Autodesk Fusion 360 part; units mm, degrees
(part 5 of 6)
  arc A937 (93.55, -32.3196) -> (93.5061, -32.1633) centre (93.25, -32.3196) ccw
  arc A938 (94.1933, -31.4761) -> (93.5061, -32.1633) centre (93.9328, -31.9028) ccw
  arc A939 (94.1933, -31.4761) -> (94.3496, -31.52) centre (94.3496, -31.22) ccw
  line L528 (94.3496, -31.52) -> (95.25, -31.52)
  line L529 (95.25, -31.52) -> (96.1504, -31.52)
  arc A940 (96.1504, -31.52) -> (96.3067, -31.4761) centre (96.1503, -31.22) ccw
  arc A941 (96.9939, -32.1633) -> (96.3067, -31.4761) centre (96.5672, -31.9028) ccw
  arc A942 (96.9939, -32.1633) -> (96.95, -32.3196) centre (97.2501, -32.3197) ccw
  line L530 (96.95, -32.3196) -> (96.95, -33.02)
  line L531 (96.95, -33.02) -> (96.95, -33.7204)
  arc A943 (96.95, -33.7204) -> (96.9939, -33.8767) centre (97.25, -33.7203) ccw
  circle A944 centre (78.4225, -19.3675) radius 1.5
  circle A945 centre (59.3725, -19.3675) radius 1.5
  arc A946 (77.2567, -34.5639) -> (77.9439, -33.8767) centre (77.5172, -34.1372) ccw
  arc A947 (77.2567, -34.5639) -> (77.1004, -34.52) centre (77.1004, -34.8197) ccw
  line L532 (77.1004, -34.52) -> (76.2, -34.52)
  line L533 (76.2, -34.52) -> (75.2996, -34.52)
  arc A948 (75.2996, -34.52) -> (75.1433, -34.5639) centre (75.2996, -34.82) ccw
  arc A949 (74.4561, -33.8767) -> (75.1433, -34.5639) centre (74.8828, -34.1372) ccw
  arc A950 (74.4561, -33.8767) -> (74.5, -33.7204) centre (74.2, -33.7204) ccw
  line L534 (74.5, -33.7204) -> (74.5, -33.02)
  line L535 (74.5, -33.02) -> (74.5, -32.3196)
  arc A951 (74.5, -32.3196) -> (74.4561, -32.1633) centre (74.2, -32.3196) ccw
  arc A952 (75.1433, -31.4761) -> (74.4561, -32.1633) centre (74.8828, -31.9028) ccw
  arc A953 (75.1433, -31.4761) -> (75.2996, -31.52) centre (75.2996, -31.22) ccw
  line L536 (75.2996, -31.52) -> (76.2, -31.52)
  line L537 (76.2, -31.52) -> (77.1004, -31.52)
  arc A954 (77.1004, -31.52) -> (77.2567, -31.4761) centre (77.1003, -31.22) ccw
  arc A955 (77.9439, -32.1633) -> (77.2567, -31.4761) centre (77.5172, -31.9028) ccw
  arc A956 (77.9439, -32.1633) -> (77.9, -32.3196) centre (78.2001, -32.3197) ccw
  line L538 (77.9, -32.3196) -> (77.9, -33.02)
  line L539 (77.9, -33.02) -> (77.9, -33.7204)
  arc A957 (77.9, -33.7204) -> (77.9439, -33.8767) centre (78.2, -33.7203) ccw
  arc A958 (58.2067, -34.5639) -> (58.8939, -33.8767) centre (58.4672, -34.1372) ccw
  arc A959 (58.2067, -34.5639) -> (58.0504, -34.52) centre (58.0504, -34.8197) ccw
  line L540 (58.0504, -34.52) -> (57.15, -34.52)
  line L541 (57.15, -34.52) -> (56.2496, -34.52)
  arc A960 (56.2496, -34.52) -> (56.0933, -34.5639) centre (56.2496, -34.82) ccw
  arc A961 (55.4061, -33.8767) -> (56.0933, -34.5639) centre (55.8328, -34.1372) ccw
  arc A962 (55.4061, -33.8767) -> (55.45, -33.7204) centre (55.15, -33.7204) ccw
  line L542 (55.45, -33.7204) -> (55.45, -33.02)
  line L543 (55.45, -33.02) -> (55.45, -32.3196)
  arc A963 (55.45, -32.3196) -> (55.4061, -32.1633) centre (55.15, -32.3196) ccw
  arc A964 (56.0933, -31.4761) -> (55.4061, -32.1633) centre (55.8328, -31.9028) ccw
  arc A965 (56.0933, -31.4761) -> (56.2496, -31.52) centre (56.2496, -31.22) ccw
  line L544 (56.2496, -31.52) -> (57.15, -31.52)
  line L545 (57.15, -31.52) -> (58.0504, -31.52)
  arc A966 (58.0504, -31.52) -> (58.2067, -31.4761) centre (58.0503, -31.22) ccw
  arc A967 (58.8939, -32.1633) -> (58.2067, -31.4761) centre (58.4672, -31.9028) ccw
  arc A968 (58.8939, -32.1633) -> (58.85, -32.3196) centre (59.1501, -32.3197) ccw
  line L546 (58.85, -32.3196) -> (58.85, -33.02)
  line L547 (58.85, -33.02) -> (58.85, -33.7204)
  arc A969 (58.85, -33.7204) -> (58.8939, -33.8767) centre (59.15, -33.7203) ccw
  circle A970 centre (124.1425, -38.1) radius 0.875
  circle A971 centre (122.8725, -40.64) radius 1.5
  circle A972 centre (119.0625, -38.1) radius 1.9939
  circle A973 centre (113.9825, -38.1) radius 0.875
  circle A974 centre (100.33, -38.1) radius 0.875
  circle A975 centre (95.25, -38.1) radius 1.9939
  circle A976 centre (90.17, -38.1) radius 0.875
  circle A977 centre (99.06, -40.64) radius 1.5
  circle A978 centre (116.5225, -43.18) radius 1.5
  circle A979 centre (128.5875, -47.625) radius 1.1
  circle A980 centre (92.71, -43.18) radius 1.5
  circle A981 centre (107.1563, -47.625) radius 1.1
  circle A982 centre (81.28, -38.1) radius 0.875
  circle A983 centre (76.2, -38.1) radius 1.9939
  circle A984 centre (71.12, -38.1) radius 0.875
  circle A985 centre (80.01, -40.64) radius 1.5
  circle A986 centre (62.23, -38.1) radius 0.875
  circle A987 centre (60.96, -40.64) radius 1.5
  circle A988 centre (57.15, -38.1) radius 1.9939
  circle A989 centre (52.07, -38.1) radius 0.875
  circle A990 centre (73.66, -43.18) radius 1.5
  circle A991 centre (54.61, -43.18) radius 1.5
  circle A992 centre (40.3225, -19.3675) radius 1.5
  circle A993 centre (21.2725, -19.3675) radius 1.5
  arc A994 (39.1567, -34.5639) -> (39.8439, -33.8767) centre (39.4172, -34.1372) ccw
  arc A995 (39.1567, -34.5639) -> (39.0004, -34.52) centre (39.0004, -34.8197) ccw
  line L548 (39.0004, -34.52) -> (38.1, -34.52)
  line L549 (38.1, -34.52) -> (37.1996, -34.52)
  arc A996 (37.1996, -34.52) -> (37.0433, -34.5639) centre (37.1996, -34.82) ccw
  arc A997 (36.3561, -33.8767) -> (37.0433, -34.5639) centre (36.7828, -34.1372) ccw
  arc A998 (36.3561, -33.8767) -> (36.4, -33.7204) centre (36.1, -33.7204) ccw
  line L550 (36.4, -33.7204) -> (36.4, -33.02)
  line L551 (36.4, -33.02) -> (36.4, -32.3196)
  arc A999 (36.4, -32.3196) -> (36.3561, -32.1633) centre (36.1, -32.3196) ccw
  arc A1000 (37.0433, -31.4761) -> (36.3561, -32.1633) centre (36.7828, -31.9028) ccw
  arc A1001 (37.0433, -31.4761) -> (37.1996, -31.52) centre (37.1996, -31.22) ccw
  line L552 (37.1996, -31.52) -> (38.1, -31.52)
  line L553 (38.1, -31.52) -> (39.0004, -31.52)
  arc A1002 (39.0004, -31.52) -> (39.1567, -31.4761) centre (39.0003, -31.22) ccw
  arc A1003 (39.8439, -32.1633) -> (39.1567, -31.4761) centre (39.4172, -31.9028) ccw
  arc A1004 (39.8439, -32.1633) -> (39.8, -32.3196) centre (40.1001, -32.3197) ccw
  line L554 (39.8, -32.3196) -> (39.8, -33.02)
  line L555 (39.8, -33.02) -> (39.8, -33.7204)
  arc A1005 (39.8, -33.7204) -> (39.8439, -33.8767) centre (40.1, -33.7203) ccw
  circle A1006 centre (26.1938, -26.1938) radius 1.1
  arc A1007 (15.3442, -34.5639) -> (16.0314, -33.8767) centre (15.6047, -34.1372) ccw
  arc A1008 (15.3442, -34.5639) -> (15.1879, -34.52) centre (15.1879, -34.8197) ccw
  line L556 (15.1879, -34.52) -> (14.2875, -34.52)
  line L557 (14.2875, -34.52) -> (13.3871, -34.52)
  arc A1009 (13.3871, -34.52) -> (13.2308, -34.5639) centre (13.3871, -34.82) ccw
  arc A1010 (12.5436, -33.8767) -> (13.2308, -34.5639) centre (12.9703, -34.1372) ccw
  arc A1011 (12.5436, -33.8767) -> (12.5875, -33.7204) centre (12.2875, -33.7204) ccw
  line L558 (12.5875, -33.7204) -> (12.5875, -33.02)
  line L559 (12.5875, -33.02) -> (12.5875, -32.3196)
  arc A1012 (12.5875, -32.3196) -> (12.5436, -32.1633) centre (12.2875, -32.3196) ccw
  arc A1013 (13.2308, -31.4761) -> (12.5436, -32.1633) centre (12.9703, -31.9028) ccw
  arc A1014 (13.2308, -31.4761) -> (13.3871, -31.52) centre (13.3871, -31.22) ccw
  line L560 (13.3871, -31.52) -> (14.2875, -31.52)
  line L561 (14.2875, -31.52) -> (15.1879, -31.52)
  arc A1015 (15.1879, -31.52) -> (15.3442, -31.4761) centre (15.1878, -31.22) ccw
  arc A1016 (16.0314, -32.1633) -> (15.3442, -31.4761) centre (15.6047, -31.9028) ccw
  arc A1017 (16.0314, -32.1633) -> (15.9875, -32.3196) centre (16.2876, -32.3197) ccw
  line L562 (15.9875, -32.3196) -> (15.9875, -33.02)
  line L563 (15.9875, -33.02) -> (15.9875, -33.7204)
  arc A1018 (15.9875, -33.7204) -> (16.0314, -33.8767) centre (16.2875, -33.7203) ccw
  circle A1019 centre (2.2225, -19.3675) radius 1.5
  circle A1020 centre (-16.8275, -19.3675) radius 1.5
  arc A1021 (-6.5064, -33.8767) -> (-5.8192, -34.5639) centre (-6.0797, -34.1372) ccw
  arc A1022 (-6.5064, -33.8767) -> (-6.4625, -33.7204) centre (-6.7625, -33.7204) ccw
  line L564 (-6.4625, -33.7204) -> (-6.4625, -33.02)
  line L565 (-6.4625, -33.02) -> (-6.4625, -32.3196)
  arc A1023 (-6.4625, -32.3196) -> (-6.5064, -32.1633) centre (-6.7625, -32.3196) ccw
  arc A1024 (-5.8192, -31.4761) -> (-6.5064, -32.1633) centre (-6.0797, -31.9028) ccw
  arc A1025 (-5.8192, -31.4761) -> (-5.6629, -31.52) centre (-5.6629, -31.22) ccw
  line L566 (-5.6629, -31.52) -> (-4.7625, -31.52)
  line L567 (-4.7625, -31.52) -> (-3.8621, -31.52)
  arc A1026 (-3.8621, -31.52) -> (-3.7058, -31.4761) centre (-3.8622, -31.22) ccw
  arc A1027 (-3.0186, -32.1633) -> (-3.7058, -31.4761) centre (-3.4453, -31.9028) ccw
  arc A1028 (-3.0186, -32.1633) -> (-3.0625, -32.3196) centre (-2.7624, -32.3197) ccw
  line L568 (-3.0625, -32.3196) -> (-3.0625, -33.02)
  line L569 (-3.0625, -33.02) -> (-3.0625, -33.7204)
  arc A1029 (-3.0625, -33.7204) -> (-3.0186, -33.8767) centre (-2.7625, -33.7203) ccw
  arc A1030 (-3.7058, -34.5639) -> (-3.0186, -33.8767) centre (-3.4453, -34.1372) ccw
  arc A1031 (-3.7058, -34.5639) -> (-3.8621, -34.52) centre (-3.8621, -34.8197) ccw
  line L570 (-3.8621, -34.52) -> (-4.7625, -34.52)
  line L571 (-4.7625, -34.52) -> (-5.6629, -34.52)
  arc A1032 (-5.6629, -34.52) -> (-5.8192, -34.5639) centre (-5.6629, -34.82) ccw
  arc A1033 (-25.5564, -33.8767) -> (-24.8692, -34.5639) centre (-25.1297, -34.1372) ccw
  arc A1034 (-25.5564, -33.8767) -> (-25.5125, -33.7204) centre (-25.8125, -33.7204) ccw
  line L572 (-25.5125, -33.7204) -> (-25.5125, -33.02)
  line L573 (-25.5125, -33.02) -> (-25.5125, -32.3196)
  arc A1035 (-25.5125, -32.3196) -> (-25.5564, -32.1633) centre (-25.8125, -32.3196) ccw
  arc A1036 (-24.8692, -31.4761) -> (-25.5564, -32.1633) centre (-25.1297, -31.9028) ccw
  arc A1037 (-24.8692, -31.4761) -> (-24.7129, -31.52) centre (-24.7129, -31.22) ccw
  line L574 (-24.7129, -31.52) -> (-23.8125, -31.52)
  line L575 (-23.8125, -31.52) -> (-22.9121, -31.52)
  arc A1038 (-22.9121, -31.52) -> (-22.7558, -31.4761) centre (-22.9122, -31.22) ccw
  arc A1039 (-22.0686, -32.1633) -> (-22.7558, -31.4761) centre (-22.4953, -31.9028) ccw
  arc A1040 (-22.0686, -32.1633) -> (-22.1125, -32.3196) centre (-21.8124, -32.3197) ccw
  line L576 (-22.1125, -32.3196) -> (-22.1125, -33.02)
  line L577 (-22.1125, -33.02) -> (-22.1125, -33.7204)
  arc A1041 (-22.1125, -33.7204) -> (-22.0686, -33.8767) centre (-21.8125, -33.7203) ccw
  arc A1042 (-22.7558, -34.5639) -> (-22.0686, -33.8767) centre (-22.4953, -34.1372) ccw
  arc A1043 (-22.7558, -34.5639) -> (-22.9121, -34.52) centre (-22.9121, -34.8197) ccw
  line L578 (-22.9121, -34.52) -> (-23.8125, -34.52)
  line L579 (-23.8125, -34.52) -> (-24.7129, -34.52)
  arc A1044 (-24.7129, -34.52) -> (-24.8692, -34.5639) centre (-24.7129, -34.82) ccw
  circle A1045 centre (43.18, -38.1) radius 0.875
  circle A1046 centre (41.91, -40.64) radius 1.5
  circle A1047 centre (38.1, -38.1) radius 1.9939
  circle A1048 centre (33.02, -38.1) radius 0.875
  circle A1049 centre (19.3675, -38.1) radius 0.875
  circle A1050 centre (14.2875, -38.1) radius 1.9939
  circle A1051 centre (18.0975, -40.64) radius 1.5
  circle A1052 centre (35.56, -43.18) radius 1.5
  circle A1053 centre (11.7475, -43.18) radius 1.5
  circle A1054 centre (26.1938, -47.625) radius 1.1
  circle A1055 centre (9.2075, -38.1) radius 0.875
  circle A1056 centre (0.3175, -38.1) radius 0.875
  circle A1057 centre (-4.7625, -38.1) radius 1.9939
  circle A1058 centre (-0.9525, -40.64) radius 1.5
  circle A1059 centre (-9.8425, -38.1) radius 0.875
  circle A1060 centre (-18.7325, -38.1) radius 0.875
  circle A1061 centre (-23.8125, -38.1) radius 1.9939
  circle A1062 centre (-20.0025, -40.64) radius 1.5
  circle A1063 centre (-7.3025, -43.18) radius 1.5
  circle A1064 centre (-26.3525, -43.18) radius 1.5
  arc A1065 (-44.6064, 8.9858) -> (-43.9192, 8.2986) centre (-44.1797, 8.7253) ccw
  arc A1066 (-44.6064, 8.9858) -> (-44.5625, 9.1421) centre (-44.8625, 9.1421) ccw
  line L580 (-44.5625, 9.1421) -> (-44.5625, 9.8425)
  line L581 (-44.5625, 9.8425) -> (-44.5625, 10.5429)
  arc A1067 (-44.5625, 10.5429) -> (-44.6064, 10.6992) centre (-44.8625, 10.5429) ccw
  arc A1068 (-43.9192, 11.3864) -> (-44.6064, 10.6992) centre (-44.1797, 10.9597) ccw
  arc A1069 (-43.9192, 11.3864) -> (-43.7629, 11.3425) centre (-43.7629, 11.6425) ccw
  line L582 (-43.7629, 11.3425) -> (-42.8625, 11.3425)
  line L583 (-42.8625, 11.3425) -> (-41.9621, 11.3425)
  arc A1070 (-41.9621, 11.3425) -> (-41.8058, 11.3864) centre (-41.9622, 11.6425) ccw
  arc A1071 (-41.1186, 10.6992) -> (-41.8058, 11.3864) centre (-41.5453, 10.9597) ccw
  arc A1072 (-41.1186, 10.6992) -> (-41.1625, 10.5429) centre (-40.8624, 10.5428) ccw
  line L584 (-41.1625, 10.5429) -> (-41.1625, 9.8425)
  line L585 (-41.1625, 9.8425) -> (-41.1625, 9.1421)
  arc A1073 (-41.1625, 9.1421) -> (-41.1186, 8.9858) centre (-40.8625, 9.1422) ccw
  arc A1074 (-41.8058, 8.2986) -> (-41.1186, 8.9858) centre (-41.5453, 8.7253) ccw
  arc A1075 (-41.8058, 8.2986) -> (-41.9621, 8.3425) centre (-41.9621, 8.0428) ccw
  line L586 (-41.9621, 8.3425) -> (-42.8625, 8.3425)
  line L587 (-42.8625, 8.3425) -> (-43.7629, 8.3425)
  arc A1076 (-43.7629, 8.3425) -> (-43.9192, 8.2986) centre (-43.7629, 8.0425) ccw
  arc A1077 (-63.6564, 8.9858) -> (-62.9692, 8.2986) centre (-63.2297, 8.7253) ccw
  arc A1078 (-63.6564, 8.9858) -> (-63.6125, 9.1421) centre (-63.9125, 9.1421) ccw
  line L588 (-63.6125, 9.1421) -> (-63.6125, 9.8425)
  line L589 (-63.6125, 9.8425) -> (-63.6125, 10.5429)
  arc A1079 (-63.6125, 10.5429) -> (-63.6564, 10.6992) centre (-63.9125, 10.5429) ccw
  arc A1080 (-62.9692, 11.3864) -> (-63.6564, 10.6992) centre (-63.2297, 10.9597) ccw
  arc A1081 (-62.9692, 11.3864) -> (-62.8129, 11.3425) centre (-62.8129, 11.6425) ccw
  line L590 (-62.8129, 11.3425) -> (-61.9125, 11.3425)
  line L591 (-61.9125, 11.3425) -> (-61.0121, 11.3425)
  arc A1082 (-61.0121, 11.3425) -> (-60.8558, 11.3864) centre (-61.0122, 11.6425) ccw
  arc A1083 (-60.1686, 10.6992) -> (-60.8558, 11.3864) centre (-60.5953, 10.9597) ccw
  arc A1084 (-60.1686, 10.6992) -> (-60.2125, 10.5429) centre (-59.9124, 10.5428) ccw
  line L592 (-60.2125, 10.5429) -> (-60.2125, 9.8425)
  line L593 (-60.2125, 9.8425) -> (-60.2125, 9.1421)
  arc A1085 (-60.2125, 9.1421) -> (-60.1686, 8.9858) centre (-59.9125, 9.1422) ccw
  arc A1086 (-60.8558, 8.2986) -> (-60.1686, 8.9858) centre (-60.5953, 8.7253) ccw
  arc A1087 (-60.8558, 8.2986) -> (-61.0121, 8.3425) centre (-61.0121, 8.0428) ccw
  line L594 (-61.0121, 8.3425) -> (-61.9125, 8.3425)
  line L595 (-61.9125, 8.3425) -> (-62.8129, 8.3425)
  arc A1088 (-62.8129, 8.3425) -> (-62.9692, 8.2986) centre (-62.8129, 8.0425) ccw
  circle A1089 centre (-28.8925, 4.7625) radius 0.875
  circle A1090 centre (-37.7825, 4.7625) radius 0.875
  circle A1091 centre (-42.8625, 4.7625) radius 1.9939
  circle A1092 centre (-47.9425, 4.7625) radius 0.875
  circle A1093 centre (-39.0525, 2.2225) radius 1.5
  circle A1094 centre (-45.4025, -0.3175) radius 1.5
  circle A1095 centre (-56.8325, 4.7625) radius 0.875
  circle A1096 centre (-58.1025, 2.2225) radius 1.5
  circle A1097 centre (-61.9125, 4.7625) radius 1.9939
  circle A1098 centre (-66.9925, 4.7625) radius 0.875
  circle A1099 centre (-64.4525, -0.3175) radius 1.5
  arc A1100 (-82.7064, 8.9858) -> (-82.0192, 8.2986) centre (-82.2797, 8.7253) ccw
  arc A1101 (-82.7064, 8.9858) -> (-82.6625, 9.1421) centre (-82.9625, 9.1421) ccw
  line L596 (-82.6625, 9.1421) -> (-82.6625, 9.8425)
  line L597 (-82.6625, 9.8425) -> (-82.6625, 10.5429)
  arc A1102 (-82.6625, 10.5429) -> (-82.7064, 10.6992) centre (-82.9625, 10.5429) ccw
  arc A1103 (-82.0192, 11.3864) -> (-82.7064, 10.6992) centre (-82.2797, 10.9597) ccw
  arc A1104 (-82.0192, 11.3864) -> (-81.8629, 11.3425) centre (-81.8629, 11.6425) ccw
  line L598 (-81.8629, 11.3425) -> (-80.9625, 11.3425)
  line L599 (-80.9625, 11.3425) -> (-80.0621, 11.3425)
  arc A1105 (-80.0621, 11.3425) -> (-79.9058, 11.3864) centre (-80.0622, 11.6425) ccw
  arc A1106 (-79.2186, 10.6992) -> (-79.9058, 11.3864) centre (-79.6453, 10.9597) ccw
  arc A1107 (-79.2186, 10.6992) -> (-79.2625, 10.5429) centre (-78.9624, 10.5428) ccw
  line L600 (-79.2625, 10.5429) -> (-79.2625, 9.8425)
  line L601 (-79.2625, 9.8425) -> (-79.2625, 9.1421)
  arc A1108 (-79.2625, 9.1421) -> (-79.2186, 8.9858) centre (-78.9625, 9.1422) ccw
  arc A1109 (-79.9058, 8.2986) -> (-79.2186, 8.9858) centre (-79.6453, 8.7253) ccw
  arc A1110 (-79.9058, 8.2986) -> (-80.0621, 8.3425) centre (-80.0621, 8.0428) ccw
  line L602 (-80.0621, 8.3425) -> (-80.9625, 8.3425)
  line L603 (-80.9625, 8.3425) -> (-81.8629, 8.3425)
  arc A1111 (-81.8629, 8.3425) -> (-82.0192, 8.2986) centre (-81.8629, 8.0425) ccw
  arc A1112 (-101.7564, 8.9858) -> (-101.0692, 8.2986) centre (-101.3297, 8.7253) ccw
  arc A1113 (-101.7564, 8.9858) -> (-101.7125, 9.1421) centre (-102.0125, 9.1421) ccw
  line L604 (-101.7125, 9.1421) -> (-101.7125, 9.8425)
  line L605 (-101.7125, 9.8425) -> (-101.7125, 10.5429)
  arc A1114 (-101.7125, 10.5429) -> (-101.7564, 10.6992) centre (-102.0125, 10.5429) ccw
  arc A1115 (-101.0692, 11.3864) -> (-101.7564, 10.6992) centre (-101.3297, 10.9597) ccw
  arc A1116 (-101.0692, 11.3864) -> (-100.9129, 11.3425) centre (-100.9129, 11.6425) ccw
  line L606 (-100.9129, 11.3425) -> (-100.0125, 11.3425)
  line L607 (-100.0125, 11.3425) -> (-99.1121, 11.3425)
  arc A1117 (-99.1121, 11.3425) -> (-98.9558, 11.3864) centre (-99.1122, 11.6425) ccw
  arc A1118 (-98.2686, 10.6992) -> (-98.9558, 11.3864) centre (-98.6953, 10.9597) ccw
  arc A1119 (-98.2686, 10.6992) -> (-98.3125, 10.5429) centre (-98.0124, 10.5428) ccw
  line L608 (-98.3125, 10.5429) -> (-98.3125, 9.8425)
  line L609 (-98.3125, 9.8425) -> (-98.3125, 9.1421)
  arc A1120 (-98.3125, 9.1421) -> (-98.2686, 8.9858) centre (-98.0125, 9.1422) ccw
  arc A1121 (-98.9558, 8.2986) -> (-98.2686, 8.9858) centre (-98.6953, 8.7253) ccw
  arc A1122 (-98.9558, 8.2986) -> (-99.1121, 8.3425) centre (-99.1121, 8.0428) ccw
  line L610 (-99.1121, 8.3425) -> (-100.0125, 8.3425)
  line L611 (-100.0125, 8.3425) -> (-100.9129, 8.3425)
  arc A1123 (-100.9129, 8.3425) -> (-101.0692, 8.2986) centre (-100.9129, 8.0425) ccw
  circle A1124 centre (-75.8825, 4.7625) radius 0.875
  circle A1125 centre (-77.1525, 2.2225) radius 1.5
  circle A1126 centre (-80.9625, 4.7625) radius 1.9939
  circle A1127 centre (-86.0425, 4.7625) radius 0.875
  circle A1128 centre (-83.5025, -0.3175) radius 1.5
  circle A1129 centre (-94.9325, 4.7625) radius 0.875
  circle A1130 centre (-96.2025, 2.2225) radius 1.5
  circle A1131 centre (-100.0125, 4.7625) radius 1.9939
  circle A1132 centre (-105.0925, 4.7625) radius 0.875
  circle A1133 centre (-102.5525, -0.3175) radius 1.5
  arc A1134 (-35.0814, -10.0642) -> (-34.3942, -10.7514) centre (-34.6547, -10.3247) ccw
  arc A1135 (-35.0814, -10.0642) -> (-35.0375, -9.9079) centre (-35.3375, -9.9079) ccw
  line L612 (-35.0375, -9.9079) -> (-35.0375, -9.2075)
  line L613 (-35.0375, -9.2075) -> (-35.0375, -8.5071)
  arc A1136 (-35.0375, -8.5071) -> (-35.0814, -8.3508) centre (-35.3375, -8.5071) ccw
  arc A1137 (-34.3942, -7.6636) -> (-35.0814, -8.3508) centre (-34.6547, -8.0903) ccw
  arc A1138 (-34.3942, -7.6636) -> (-34.2379, -7.7075) centre (-34.2379, -7.4075) ccw
  line L614 (-34.2379, -7.7075) -> (-33.3375, -7.7075)
  line L615 (-33.3375, -7.7075) -> (-32.4371, -7.7075)
  arc A1139 (-32.4371, -7.7075) -> (-32.2808, -7.6636) centre (-32.4372, -7.4075) ccw
  arc A1140 (-31.5936, -8.3508) -> (-32.2808, -7.6636) centre (-32.0203, -8.0903) ccw
  arc A1141 (-31.5936, -8.3508) -> (-31.6375, -8.5071) centre (-31.3374, -8.5072) ccw
  line L616 (-31.6375, -8.5071) -> (-31.6375, -9.2075)
  line L617 (-31.6375, -9.2075) -> (-31.6375, -9.9079)
  arc A1142 (-31.6375, -9.9079) -> (-31.5936, -10.0642) centre (-31.3375, -9.9078) ccw
  arc A1143 (-32.2808, -10.7514) -> (-31.5936, -10.0642) centre (-32.0203, -10.3247) ccw
  arc A1144 (-32.2808, -10.7514) -> (-32.4371, -10.7075) centre (-32.4371, -11.0072) ccw
  line L618 (-32.4371, -10.7075) -> (-33.3375, -10.7075)
  line L619 (-33.3375, -10.7075) -> (-34.2379, -10.7075)
  arc A1145 (-34.2379, -10.7075) -> (-34.3942, -10.7514) centre (-34.2379, -11.0075) ccw
  arc A1146 (-54.1314, -10.0642) -> (-53.4442, -10.7514) centre (-53.7047, -10.3247) ccw
  arc A1147 (-54.1314, -10.0642) -> (-54.0875, -9.9079) centre (-54.3875, -9.9079) ccw
  line L620 (-54.0875, -9.9079) -> (-54.0875, -9.2075)
  line L621 (-54.0875, -9.2075) -> (-54.0875, -8.5071)
  arc A1148 (-54.0875, -8.5071) -> (-54.1314, -8.3508) centre (-54.3875, -8.5071) ccw
  arc A1149 (-53.4442, -7.6636) -> (-54.1314, -8.3508) centre (-53.7047, -8.0903) ccw
  arc A1150 (-53.4442, -7.6636) -> (-53.2879, -7.7075) centre (-53.2879, -7.4075) ccw
  line L622 (-53.2879, -7.7075) -> (-52.3875, -7.7075)
  line L623 (-52.3875, -7.7075) -> (-51.4871, -7.7075)
  arc A1151 (-51.4871, -7.7075) -> (-51.3308, -7.6636) centre (-51.4872, -7.4075) ccw
  arc A1152 (-50.6436, -8.3508) -> (-51.3308, -7.6636) centre (-51.0703, -8.0903) ccw
  arc A1153 (-50.6436, -8.3508) -> (-50.6875, -8.5071) centre (-50.3874, -8.5072) ccw
  line L624 (-50.6875, -8.5071) -> (-50.6875, -9.2075)
  line L625 (-50.6875, -9.2075) -> (-50.6875, -9.9079)
  arc A1154 (-50.6875, -9.9079) -> (-50.6436, -10.0642) centre (-50.3875, -9.9078) ccw
  arc A1155 (-51.3308, -10.7514) -> (-50.6436, -10.0642) centre (-51.0703, -10.3247) ccw
  arc A1156 (-51.3308, -10.7514) -> (-51.4871, -10.7075) centre (-51.4871, -11.0072) ccw
  line L626 (-51.4871, -10.7075) -> (-52.3875, -10.7075)
  line L627 (-52.3875, -10.7075) -> (-53.2879, -10.7075)
  arc A1157 (-53.2879, -10.7075) -> (-53.4442, -10.7514) centre (-53.2879, -11.0075) ccw
  circle A1158 centre (-33.3375, -14.2875) radius 1.9939
  circle A1159 centre (-38.4175, -14.2875) radius 0.875
  circle A1160 centre (-29.5275, -16.8275) radius 1.5
  circle A1161 centre (-47.3075, -14.2875) radius 0.875
  circle A1162 centre (-52.3875, -14.2875) radius 1.9939
  circle A1163 centre (-57.4675, -14.2875) radius 0.875
  circle A1164 centre (-48.5775, -16.8275) radius 1.5
  circle A1165 centre (-66.3575, -14.2875) radius 0.875
  circle A1166 centre (-67.6275, -16.8275) radius 1.5
  arc A1167 (-73.1814, -10.0642) -> (-72.4942, -10.7514) centre (-72.7547, -10.3247) ccw
  arc A1168 (-73.1814, -10.0642) -> (-73.1375, -9.9079) centre (-73.4375, -9.9079) ccw
  line L628 (-73.1375, -9.9079) -> (-73.1375, -9.2075)
  line L629 (-73.1375, -9.2075) -> (-73.1375, -8.5071)
  arc A1169 (-73.1375, -8.5071) -> (-73.1814, -8.3508) centre (-73.4375, -8.5071) ccw
  arc A1170 (-72.4942, -7.6636) -> (-73.1814, -8.3508) centre (-72.7547, -8.0903) ccw
  arc A1171 (-72.4942, -7.6636) -> (-72.3379, -7.7075) centre (-72.3379, -7.4075) ccw
  line L630 (-72.3379, -7.7075) -> (-71.4375, -7.7075)
  line L631 (-71.4375, -7.7075) -> (-70.5371, -7.7075)
  arc A1172 (-70.5371, -7.7075) -> (-70.3808, -7.6636) centre (-70.5372, -7.4075) ccw
  arc A1173 (-69.6936, -8.3508) -> (-70.3808, -7.6636) centre (-70.1203, -8.0903) ccw
  arc A1174 (-69.6936, -8.3508) -> (-69.7375, -8.5071) centre (-69.4374, -8.5072) ccw
  line L632 (-69.7375, -8.5071) -> (-69.7375, -9.2075)
  line L633 (-69.7375, -9.2075) -> (-69.7375, -9.9079)
  arc A1175 (-69.7375, -9.9079) -> (-69.6936, -10.0642) centre (-69.4375, -9.9078) ccw
  arc A1176 (-70.3808, -10.7514) -> (-69.6936, -10.0642) centre (-70.1203, -10.3247) ccw
  arc A1177 (-70.3808, -10.7514) -> (-70.5371, -10.7075) centre (-70.5371, -11.0072) ccw
  line L634 (-70.5371, -10.7075) -> (-71.4375, -10.7075)
  line L635 (-71.4375, -10.7075) -> (-72.3379, -10.7075)
  arc A1178 (-72.3379, -10.7075) -> (-72.4942, -10.7514) centre (-72.3379, -11.0075) ccw
  arc A1179 (-92.2314, -10.0642) -> (-91.5442, -10.7514) centre (-91.8047, -10.3247) ccw
  arc A1180 (-92.2314, -10.0642) -> (-92.1875, -9.9079) centre (-92.4875, -9.9079) ccw
  line L636 (-92.1875, -9.9079) -> (-92.1875, -9.2075)
  line L637 (-92.1875, -9.2075) -> (-92.1875, -8.5071)
  arc A1181 (-92.1875, -8.5071) -> (-92.2314, -8.3508) centre (-92.4875, -8.5071) ccw
  arc A1182 (-91.5442, -7.6636) -> (-92.2314, -8.3508) centre (-91.8047, -8.0903) ccw
  arc A1183 (-91.5442, -7.6636) -> (-91.3879, -7.7075) centre (-91.3879, -7.4075) ccw
  line L638 (-91.3879, -7.7075) -> (-90.4875, -7.7075)
  line L639 (-90.4875, -7.7075) -> (-89.5871, -7.7075)
  arc A1184 (-89.5871, -7.7075) -> (-89.4308, -7.6636) centre (-89.5872, -7.4075) ccw
  arc A1185 (-88.7436, -8.3508) -> (-89.4308, -7.6636) centre (-89.1703, -8.0903) ccw
  arc A1186 (-88.7436, -8.3508) -> (-88.7875, -8.5071) centre (-88.4874, -8.5072) ccw
  line L640 (-88.7875, -8.5071) -> (-88.7875, -9.2075)
  line L641 (-88.7875, -9.2075) -> (-88.7875, -9.9079)
  arc A1187 (-88.7875, -9.9079) -> (-88.7436, -10.0642) centre (-88.4875, -9.9078) ccw
  arc A1188 (-89.4308, -10.7514) -> (-88.7436, -10.0642) centre (-89.1703, -10.3247) ccw
  arc A1189 (-89.4308, -10.7514) -> (-89.5871, -10.7075) centre (-89.5871, -11.0072) ccw
  line L642 (-89.5871, -10.7075) -> (-90.4875, -10.7075)
  line L643 (-90.4875, -10.7075) -> (-91.3879, -10.7075)
  arc A1190 (-91.3879, -10.7075) -> (-91.5442, -10.7514) centre (-91.3879, -11.0075) ccw
  circle A1191 centre (-71.4375, -14.2875) radius 1.9939
  circle A1192 centre (-76.5175, -14.2875) radius 0.875
  circle A1193 centre (-85.4075, -14.2875) radius 0.875
  circle A1194 centre (-86.6775, -16.8275) radius 1.5
  circle A1195 centre (-90.4875, -14.2875) radius 1.9939
  circle A1196 centre (-95.5675, -14.2875) radius 0.875
  circle A1197 centre (-104.4575, -14.2875) radius 0.875
  circle A1198 centre (-105.7275, -16.8275) radius 1.5
  arc A1199 (-120.8064, 8.9858) -> (-120.1192, 8.2986) centre (-120.3797, 8.7253) ccw
  arc A1200 (-120.8064, 8.9858) -> (-120.7625, 9.1421) centre (-121.0625, 9.1421) ccw
  line L644 (-120.7625, 9.1421) -> (-120.7625, 9.8425)
  line L645 (-120.7625, 9.8425) -> (-120.7625, 10.5429)
  arc A1201 (-120.7625, 10.5429) -> (-120.8064, 10.6992) centre (-121.0625, 10.5429) ccw
  arc A1202 (-120.1192, 11.3864) -> (-120.8064, 10.6992) centre (-120.3797, 10.9597) ccw
  arc A1203 (-120.1192, 11.3864) -> (-119.9629, 11.3425) centre (-119.9629, 11.6425) ccw
  line L646 (-119.9629, 11.3425) -> (-119.0625, 11.3425)
  line L647 (-119.0625, 11.3425) -> (-118.1621, 11.3425)
  arc A1204 (-118.1621, 11.3425) -> (-118.0058, 11.3864) centre (-118.1622, 11.6425) ccw
  arc A1205 (-117.3186, 10.6992) -> (-118.0058, 11.3864) centre (-117.7453, 10.9597) ccw
  arc A1206 (-117.3186, 10.6992) -> (-117.3625, 10.5429) centre (-117.0624, 10.5428) ccw
  line L648 (-117.3625, 10.5429) -> (-117.3625, 9.8425)
  line L649 (-117.3625, 9.8425) -> (-117.3625, 9.1421)
  arc A1207 (-117.3625, 9.1421) -> (-117.3186, 8.9858) centre (-117.0625, 9.1422) ccw
  arc A1208 (-118.0058, 8.2986) -> (-117.3186, 8.9858) centre (-117.7453, 8.7253) ccw
  arc A1209 (-118.0058, 8.2986) -> (-118.1621, 8.3425) centre (-118.1621, 8.0428) ccw
  line L650 (-118.1621, 8.3425) -> (-119.0625, 8.3425)
  line L651 (-119.0625, 8.3425) -> (-119.9629, 8.3425)
  arc A1210 (-119.9629, 8.3425) -> (-120.1192, 8.2986) centre (-119.9629, 8.0425) ccw
  arc A1211 (-144.6189, 8.9858) -> (-143.9317, 8.2986) centre (-144.1922, 8.7253) ccw
  arc A1212 (-144.6189, 8.9858) -> (-144.575, 9.1421) centre (-144.875, 9.1421) ccw
  line L652 (-144.575, 9.1421) -> (-144.575, 9.8425)
  line L653 (-144.575, 9.8425) -> (-144.575, 10.5429)
  arc A1213 (-144.575, 10.5429) -> (-144.6189, 10.6992) centre (-144.875, 10.5429) ccw
  arc A1214 (-143.9317, 11.3864) -> (-144.6189, 10.6992) centre (-144.1922, 10.9597) ccw
  arc A1215 (-143.9317, 11.3864) -> (-143.7754, 11.3425) centre (-143.7754, 11.6425) ccw
  line L654 (-143.7754, 11.3425) -> (-142.875, 11.3425)
  line L655 (-142.875, 11.3425) -> (-141.9746, 11.3425)
  arc A1216 (-141.9746, 11.3425) -> (-141.8183, 11.3864) centre (-141.9747, 11.6425) ccw
  arc A1217 (-141.1311, 10.6992) -> (-141.8183, 11.3864) centre (-141.5578, 10.9597) ccw
  arc A1218 (-141.1311, 10.6992) -> (-141.175, 10.5429) centre (-140.8749, 10.5428) ccw
  line L656 (-141.175, 10.5429) -> (-141.175, 9.8425)
  line L657 (-141.175, 9.8425) -> (-141.175, 9.1421)
  arc A1219 (-141.175, 9.1421) -> (-141.1311, 8.9858) centre (-140.875, 9.1422) ccw
  arc A1220 (-141.8183, 8.2986) -> (-141.1311, 8.9858) centre (-141.5578, 8.7253) ccw
  arc A1221 (-141.8183, 8.2986) -> (-141.9746, 8.3425) centre (-141.9746, 8.0428) ccw
  line L658 (-141.9746, 8.3425) -> (-142.875, 8.3425)
  line L659 (-142.875, 8.3425) -> (-143.7754, 8.3425)
  arc A1222 (-143.7754, 8.3425) -> (-143.9317, 8.2986) centre (-143.7754, 8.0425) ccw
  circle A1223 centre (-113.9825, 4.7625) radius 0.875
  circle A1224 centre (-115.2525, 2.2225) radius 1.5
  circle A1225 centre (-119.0625, 4.7625) radius 1.9939
  circle A1226 centre (-124.1425, 4.7625) radius 0.875
  circle A1227 centre (-121.6025, -0.3175) radius 1.5
  circle A1228 centre (-137.795, 4.7625) radius 0.875
  circle A1229 centre (-142.875, 4.7625) radius 1.9939
  circle A1230 centre (-139.065, 2.2225) radius 1.5
  circle A1231 centre (-145.415, -0.3175) radius 1.5
  arc A1232 (-177.9564, 8.9858) -> (-177.2692, 8.2986) centre (-177.5297, 8.7253) ccw
  arc A1233 (-177.9564, 8.9858) -> (-177.9125, 9.1421) centre (-178.2125, 9.1421) ccw
  line L660 (-177.9125, 9.1421) -> (-177.9125, 9.8425)
  line L661 (-177.9125, 9.8425) -> (-177.9125, 10.5429)
  arc A1234 (-177.9125, 10.5429) -> (-177.9564, 10.6992) centre (-178.2125, 10.5429) ccw
  arc A1235 (-177.2692, 11.3864) -> (-177.9564, 10.6992) centre (-177.5297, 10.9597) ccw
  arc A1236 (-177.2692, 11.3864) -> (-177.1129, 11.3425) centre (-177.1129, 11.6425) ccw
  line L662 (-177.1129, 11.3425) -> (-176.2125, 11.3425)
  line L663 (-176.2125, 11.3425) -> (-175.3121, 11.3425)
  arc A1237 (-175.3121, 11.3425) -> (-175.1558, 11.3864) centre (-175.3122, 11.6425) ccw
  arc A1238 (-174.4686, 10.6992) -> (-175.1558, 11.3864) centre (-174.8953, 10.9597) ccw
  arc A1239 (-174.4686, 10.6992) -> (-174.5125, 10.5429) centre (-174.2124, 10.5428) ccw
  line L664 (-174.5125, 10.5429) -> (-174.5125, 9.8425)
  line L665 (-174.5125, 9.8425) -> (-174.5125, 9.1421)
  arc A1240 (-174.5125, 9.1421) -> (-174.4686, 8.9858) centre (-174.2125, 9.1422) ccw
  arc A1241 (-175.1558, 8.2986) -> (-174.4686, 8.9858) centre (-174.8953, 8.7253) ccw
  arc A1242 (-175.1558, 8.2986) -> (-175.3121, 8.3425) centre (-175.3121, 8.0428) ccw
  line L666 (-175.3121, 8.3425) -> (-176.2125, 8.3425)
  line L667 (-176.2125, 8.3425) -> (-177.1129, 8.3425)
  arc A1243 (-177.1129, 8.3425) -> (-177.2692, 8.2986) centre (-177.1129, 8.0425) ccw
  circle A1244 centre (-147.955, 4.7625) radius 0.875
  circle A1245 centre (-171.1325, 4.7625) radius 0.875
  circle A1246 centre (-176.2125, 4.7625) radius 1.9939
  circle A1247 centre (-172.4025, 2.2225) radius 1.5
  circle A1248 centre (-181.2925, 4.7625) radius 0.875
  circle A1249 centre (-178.7525, -0.3175) radius 1.5
  arc A1250 (-111.2814, -10.0642) -> (-110.5942, -10.7514) centre (-110.8547, -10.3247) ccw
  arc A1251 (-111.2814, -10.0642) -> (-111.2375, -9.9079) centre (-111.5375, -9.9079) ccw
  line L668 (-111.2375, -9.9079) -> (-111.2375, -9.2075)
  line L669 (-111.2375, -9.2075) -> (-111.2375, -8.5071)
  arc A1252 (-111.2375, -8.5071) -> (-111.2814, -8.3508) centre (-111.5375, -8.5071) ccw
  arc A1253 (-110.5942, -7.6636) -> (-111.2814, -8.3508) centre (-110.8547, -8.0903) ccw
  arc A1254 (-110.5942, -7.6636) -> (-110.4379, -7.7075) centre (-110.4379, -7.4075) ccw
  line L670 (-110.4379, -7.7075) -> (-109.5375, -7.7075)
  line L671 (-109.5375, -7.7075) -> (-108.6371, -7.7075)
  arc A1255 (-108.6371, -7.7075) -> (-108.4808, -7.6636) centre (-108.6372, -7.4075) ccw
  arc A1256 (-107.7936, -8.3508) -> (-108.4808, -7.6636) centre (-108.2203, -8.0903) ccw
  arc A1257 (-107.7936, -8.3508) -> (-107.8375, -8.5071) centre (-107.5374, -8.5072) ccw
  line L672 (-107.8375, -8.5071) -> (-107.8375, -9.2075)
  line L673 (-107.8375, -9.2075) -> (-107.8375, -9.9079)
  arc A1258 (-107.8375, -9.9079) -> (-107.7936, -10.0642) centre (-107.5375, -9.9078) ccw
  arc A1259 (-108.4808, -10.7514) -> (-107.7936, -10.0642) centre (-108.2203, -10.3247) ccw
  arc A1260 (-108.4808, -10.7514) -> (-108.6371, -10.7075) centre (-108.6371, -11.0072) ccw
  line L674 (-108.6371, -10.7075) -> (-109.5375, -10.7075)
  line L675 (-109.5375, -10.7075) -> (-110.4379, -10.7075)
  arc A1261 (-110.4379, -10.7075) -> (-110.5942, -10.7514) centre (-110.4379, -11.0075) ccw
  arc A1262 (-139.8564, -10.0642) -> (-139.1692, -10.7514) centre (-139.4297, -10.3247) ccw
  arc A1263 (-139.8564, -10.0642) -> (-139.8125, -9.9079) centre (-140.1125, -9.9079) ccw
  line L676 (-139.8125, -9.9079) -> (-139.8125, -9.2075)
  line L677 (-139.8125, -9.2075) -> (-139.8125, -8.5071)
  arc A1264 (-139.8125, -8.5071) -> (-139.8564, -8.3508) centre (-140.1125, -8.5071) ccw
  arc A1265 (-139.1692, -7.6636) -> (-139.8564, -8.3508) centre (-139.4297, -8.0903) ccw
  arc A1266 (-139.1692, -7.6636) -> (-139.0129, -7.7075) centre (-139.0129, -7.4075) ccw
  line L678 (-139.0129, -7.7075) -> (-138.1125, -7.7075)
  line L679 (-138.1125, -7.7075) -> (-137.2121, -7.7075)
  arc A1267 (-137.2121, -7.7075) -> (-137.0558, -7.6636) centre (-137.2122, -7.4075) ccw
  arc A1268 (-136.3686, -8.3508) -> (-137.0558, -7.6636) centre (-136.7953, -8.0903) ccw
  arc A1269 (-136.3686, -8.3508) -> (-136.4125, -8.5071) centre (-136.1124, -8.5072) ccw
  line L680 (-136.4125, -8.5071) -> (-136.4125, -9.2075)
  line L681 (-136.4125, -9.2075) -> (-136.4125, -9.9079)
  arc A1270 (-136.4125, -9.9079) -> (-136.3686, -10.0642) centre (-136.1125, -9.9078) ccw
  arc A1271 (-137.0558, -10.7514) -> (-136.3686, -10.0642) centre (-136.7953, -10.3247) ccw
  arc A1272 (-137.0558, -10.7514) -> (-137.2121, -10.7075) centre (-137.2121, -11.0072) ccw
  line L682 (-137.2121, -10.7075) -> (-138.1125, -10.7075)
  line L683 (-138.1125, -10.7075) -> (-139.0129, -10.7075)
  arc A1273 (-139.0129, -10.7075) -> (-139.1692, -10.7514) centre (-139.0129, -11.0075) ccw
  circle A1274 centre (-109.5375, -14.2875) radius 1.9939
  circle A1275 centre (-114.6175, -14.2875) radius 0.875
  circle A1276 centre (-133.0325, -14.2875) radius 0.875
  circle A1277 centre (-134.3025, -16.8275) radius 1.5
  circle A1278 centre (-138.1125, -14.2875) radius 1.9939
  circle A1279 centre (-143.1925, -14.2875) radius 0.875
  circle A1280 centre (-161.925, -4.7625) radius 1.1
  arc A1281 (-175.5625, -9.4375) -> (-175.5625, -7.9375) centre (-175.5625, -8.6875) ccw
  line L684 (-175.5625, -9.4375) -> (-176.8625, -9.4375)
  arc A1282 (-176.8625, -7.9375) -> (-176.8625, -9.4375) centre (-176.8625, -8.6875) ccw
  line L685 (-176.8625, -7.9375) -> (-175.5625, -7.9375)
  circle A1283 centre (-169.2125, -11.7875) radius 0.5
  circle A1284 centre (-183.7125, -11.7875) radius 0.5
  circle A1285 centre (-176.2125, -14.2875) radius 1.05
  circle A1286 centre (-169.2125, -16.7875) radius 0.5
  arc A1287 (-180.4125, -15.0875) -> (-180.4125, -13.4875) centre (-180.4125, -14.2875) ccw
  line L686 (-180.4125, -15.0875) -> (-181.0125, -15.0875)
  arc A1288 (-181.0125, -13.4875) -> (-181.0125, -15.0875) centre (-181.0125, -14.2875) ccw
  line L687 (-181.0125, -13.4875) -> (-180.4125, -13.4875)
  circle A1289 centre (-183.7125, -14.2875) radius 0.5
  circle A1290 centre (-183.7125, -16.7875) radius 0.5
  circle A1291 centre (-35.8775, -19.3675) radius 1.5
  circle A1292 centre (-54.9275, -19.3675) radius 1.5
  arc A1293 (-44.6064, -33.8767) -> (-43.9192, -34.5639) centre (-44.1797, -34.1372) ccw
  arc A1294 (-44.6064, -33.8767) -> (-44.5625, -33.7204) centre (-44.8625, -33.7204) ccw
  line L688 (-44.5625, -33.7204) -> (-44.5625, -33.02)
  line L689 (-44.5625, -33.02) -> (-44.5625, -32.3196)
  arc A1295 (-44.5625, -32.3196) -> (-44.6064, -32.1633) centre (-44.8625, -32.3196) ccw
  arc A1296 (-43.9192, -31.4761) -> (-44.6064, -32.1633) centre (-44.1797, -31.9028) ccw
  arc A1297 (-43.9192, -31.4761) -> (-43.7629, -31.52) centre (-43.7629, -31.22) ccw
  line L690 (-43.7629, -31.52) -> (-42.8625, -31.52)
  line L691 (-42.8625, -31.52) -> (-41.9621, -31.52)
  arc A1298 (-41.9621, -31.52) -> (-41.8058, -31.4761) centre (-41.9622, -31.22) ccw
  arc A1299 (-41.1186, -32.1633) -> (-41.8058, -31.4761) centre (-41.5453, -31.9028) ccw
  arc A1300 (-41.1186, -32.1633) -> (-41.1625, -32.3196) centre (-40.8624, -32.3197) ccw
  line L692 (-41.1625, -32.3196) -> (-41.1625, -33.02)
  line L693 (-41.1625, -33.02) -> (-41.1625, -33.7204)
  arc A1301 (-41.1625, -33.7204) -> (-41.1186, -33.8767) centre (-40.8625, -33.7203) ccw
  arc A1302 (-41.8058, -34.5639) -> (-41.1186, -33.8767) centre (-41.5453, -34.1372) ccw
  arc A1303 (-41.8058, -34.5639) -> (-41.9621, -34.52) centre (-41.9621, -34.8197) ccw
  line L694 (-41.9621, -34.52) -> (-42.8625, -34.52)
  line L695 (-42.8625, -34.52) -> (-43.7629, -34.52)
  arc A1304 (-43.7629, -34.52) -> (-43.9192, -34.5639) centre (-43.7629, -34.82) ccw
  circle A1305 centre (-54.7687, -26.1938) radius 1.1
  arc A1306 (-68.4189, -33.8767) -> (-67.7317, -34.5639) centre (-67.9922, -34.1372) ccw
  arc A1307 (-68.4189, -33.8767) -> (-68.375, -33.7204) centre (-68.675, -33.7204) ccw
  line L696 (-68.375, -33.7204) -> (-68.375, -33.02)
  line L697 (-68.375, -33.02) -> (-68.375, -32.3196)
  arc A1308 (-68.375, -32.3196) -> (-68.4189, -32.1633) centre (-68.675, -32.3196) ccw
  arc A1309 (-67.7317, -31.4761) -> (-68.4189, -32.1633) centre (-67.9922, -31.9028) ccw
  arc A1310 (-67.7317, -31.4761) -> (-67.5754, -31.52) centre (-67.5754, -31.22) ccw
  line L698 (-67.5754, -31.52) -> (-66.675, -31.52)
  line L699 (-66.675, -31.52) -> (-65.7746, -31.52)
  arc A1311 (-65.7746, -31.52) -> (-65.6183, -31.4761) centre (-65.7747, -31.22) ccw
  arc A1312 (-64.9311, -32.1633) -> (-65.6183, -31.4761) centre (-65.3578, -31.9028) ccw
  arc A1313 (-64.9311, -32.1633) -> (-64.975, -32.3196) centre (-64.6749, -32.3197) ccw
  line L700 (-64.975, -32.3196) -> (-64.975, -33.02)
  line L701 (-64.975, -33.02) -> (-64.975, -33.7204)
  arc A1314 (-64.975, -33.7204) -> (-64.9311, -33.8767) centre (-64.675, -33.7203) ccw
  arc A1315 (-65.6183, -34.5639) -> (-64.9311, -33.8767) centre (-65.3578, -34.1372) ccw
  arc A1316 (-65.6183, -34.5639) -> (-65.7746, -34.52) centre (-65.7746, -34.8197) ccw
  line L702 (-65.7746, -34.52) -> (-66.675, -34.52)
  line L703 (-66.675, -34.52) -> (-67.5754, -34.52)
  arc A1317 (-67.5754, -34.52) -> (-67.7317, -34.5639) centre (-67.5754, -34.82) ccw
  circle A1318 centre (-73.9775, -19.3675) radius 1.5
  circle A1319 centre (-93.0275, -19.3675) radius 1.5
  arc A1320 (-87.4689, -33.8767) -> (-86.7817, -34.5639) centre (-87.0422, -34.1372) ccw
  arc A1321 (-87.4689, -33.8767) -> (-87.425, -33.7204) centre (-87.725, -33.7204) ccw
  line L704 (-87.425, -33.7204) -> (-87.425, -33.02)
  line L705 (-87.425, -33.02) -> (-87.425, -32.3196)
  arc A1322 (-87.425, -32.3196) -> (-87.4689, -32.1633) centre (-87.725, -32.3196) ccw
  arc A1323 (-86.7817, -31.4761) -> (-87.4689, -32.1633) centre (-87.0422, -31.9028) ccw
  arc A1324 (-86.7817, -31.4761) -> (-86.6254, -31.52) centre (-86.6254, -31.22) ccw
  line L706 (-86.6254, -31.52) -> (-85.725, -31.52)
  line L707 (-85.725, -31.52) -> (-84.8246, -31.52)
  arc A1325 (-84.8246, -31.52) -> (-84.6683, -31.4761) centre (-84.8247, -31.22) ccw
  arc A1326 (-83.9811, -32.1633) -> (-84.6683, -31.4761) centre (-84.4078, -31.9028) ccw
  arc A1327 (-83.9811, -32.1633) -> (-84.025, -32.3196) centre (-83.7249, -32.3197) ccw
  line L708 (-84.025, -32.3196) -> (-84.025, -33.02)
  line L709 (-84.025, -33.02) -> (-84.025, -33.7204)
  arc A1328 (-84.025, -33.7204) -> (-83.9811, -33.8767) centre (-83.725, -33.7203) ccw
  arc A1329 (-84.6683, -34.5639) -> (-83.9811, -33.8767) centre (-84.4078, -34.1372) ccw
  arc A1330 (-84.6683, -34.5639) -> (-84.8246, -34.52) centre (-84.8246, -34.8197) ccw
  line L710 (-84.8246, -34.52) -> (-85.725, -34.52)
  line L711 (-85.725, -34.52) -> (-86.6254, -34.52)
  arc A1331 (-86.6254, -34.52) -> (-86.7817, -34.5639) centre (-86.6254, -34.82) ccw
  arc A1332 (-106.5189, -33.8767) -> (-105.8317, -34.5639) centre (-106.0922, -34.1372) ccw
  arc A1333 (-106.5189, -33.8767) -> (-106.475, -33.7204) centre (-106.775, -33.7204) ccw
  line L712 (-106.475, -33.7204) -> (-106.475, -33.02)
  line L713 (-106.475, -33.02) -> (-106.475, -32.3196)
  arc A1334 (-106.475, -32.3196) -> (-106.5189, -32.1633) centre (-106.775, -32.3196) ccw
  arc A1335 (-105.8317, -31.4761) -> (-106.5189, -32.1633) centre (-106.0922, -31.9028) ccw
  arc A1336 (-105.8317, -31.4761) -> (-105.6754, -31.52) centre (-105.6754, -31.22) ccw
  line L714 (-105.6754, -31.52) -> (-104.775, -31.52)
  line L715 (-104.775, -31.52) -> (-103.8746, -31.52)
  arc A1337 (-103.8746, -31.52) -> (-103.7183, -31.4761) centre (-103.8747, -31.22) ccw
  arc A1338 (-103.0311, -32.1633) -> (-103.7183, -31.4761) centre (-103.4578, -31.9028) ccw
  arc A1339 (-103.0311, -32.1633) -> (-103.075, -32.3196) centre (-102.7749, -32.3197) ccw
  line L716 (-103.075, -32.3196) -> (-103.075, -33.02)
  line L717 (-103.075, -33.02) -> (-103.075, -33.7204)
  arc A1340 (-103.075, -33.7204) -> (-103.0311, -33.8767) centre (-102.775, -33.7203) ccw
  arc A1341 (-103.7183, -34.5639) -> (-103.0311, -33.8767) centre (-103.4578, -34.1372) ccw
  arc A1342 (-103.7183, -34.5639) -> (-103.8746, -34.52) centre (-103.8746, -34.8197) ccw
  line L718 (-103.8746, -34.52) -> (-104.775, -34.52)
  line L719 (-104.775, -34.52) -> (-105.6754, -34.52)
  arc A1343 (-105.6754, -34.52) -> (-105.8317, -34.5639) centre (-105.6754, -34.82) ccw
  circle A1344 centre (-28.8925, -38.1) radius 0.875
  circle A1345 centre (-37.7825, -38.1) radius 0.875
  circle A1346 centre (-42.8625, -38.1) radius 1.9939
  circle A1347 centre (-47.9425, -38.1) radius 0.875
  circle A1348 centre (-39.0525, -40.64) radius 1.5
  circle A1349 centre (-61.595, -38.1) radius 0.875
  circle A1350 centre (-66.675, -38.1) radius 1.9939
  circle A1351 centre (-62.865, -40.64) radius 1.5
  circle A1352 centre (-45.4025, -43.18) radius 1.5
  circle A1353 centre (-54.7687, -47.625) radius 1.1
  circle A1354 centre (-71.755, -38.1) radius 0.875
  circle A1355 centre (-80.645, -38.1) radius 0.875
  circle A1356 centre (-85.725, -38.1) radius 1.9939
  circle A1357 centre (-81.915, -40.64) radius 1.5
  circle A1358 centre (-90.805, -38.1) radius 0.875
  circle A1359 centre (-99.695, -38.1) radius 0.875
  circle A1360 centre (-104.775, -38.1) radius 1.9939
  circle A1361 centre (-100.965, -40.64) radius 1.5
  circle A1362 centre (-69.215, -43.18) radius 1.5
  circle A1363 centre (-88.265, -43.18) radius 1.5
  circle A1364 centre (-107.315, -43.18) radius 1.5
  circle A1365 centre (-112.0775, -19.3675) radius 1.5
  circle A1366 centre (-140.6525, -19.3675) radius 1.5
  circle A1367 centre (-138.0838, -24.5) radius 0.5
  circle A1368 centre (-140.6238, -24.5) radius 0.5
  circle A1369 centre (-143.1637, -24.5) radius 0.5
  circle A1370 centre (-145.7038, -24.5) radius 0.5
  arc A1371 (-125.5689, -33.8767) -> (-124.8817, -34.5639) centre (-125.1422, -34.1372) ccw
  arc A1372 (-125.5689, -33.8767) -> (-125.525, -33.7204) centre (-125.825, -33.7204) ccw
  line L720 (-125.525, -33.7204) -> (-125.525, -33.02)
  line L721 (-125.525, -33.02) -> (-125.525, -32.3196)
  arc A1373 (-125.525, -32.3196) -> (-125.5689, -32.1633) centre (-125.825, -32.3196) ccw
  arc A1374 (-124.8817, -31.4761) -> (-125.5689, -32.1633) centre (-125.1422, -31.9028) ccw
  arc A1375 (-124.8817, -31.4761) -> (-124.7254, -31.52) centre (-124.7254, -31.22) ccw
  line L722 (-124.7254, -31.52) -> (-123.825, -31.52)
  line L723 (-123.825, -31.52) -> (-122.9246, -31.52)
  arc A1376 (-122.9246, -31.52) -> (-122.7683, -31.4761) centre (-122.9247, -31.22) ccw
  arc A1377 (-122.0811, -32.1633) -> (-122.7683, -31.4761) centre (-122.5078, -31.9028) ccw
  arc A1378 (-122.0811, -32.1633) -> (-122.125, -32.3196) centre (-121.8249, -32.3197) ccw
  line L724 (-122.125, -32.3196) -> (-122.125, -33.02)
  line L725 (-122.125, -33.02) -> (-122.125, -33.7204)
  arc A1379 (-122.125, -33.7204) -> (-122.0811, -33.8767) centre (-121.825, -33.7203) ccw
  arc A1380 (-122.7683, -34.5639) -> (-122.0811, -33.8767) centre (-122.5078, -34.1372) ccw
  arc A1381 (-122.7683, -34.5639) -> (-122.9246, -34.52) centre (-122.9246, -34.8197) ccw
  line L726 (-122.9246, -34.52) -> (-123.825, -34.52)
  line L727 (-123.825, -34.52) -> (-124.7254, -34.52)
  arc A1382 (-124.7254, -34.52) -> (-124.8817, -34.5639) centre (-124.7254, -34.82) ccw
  circle A1383 centre (-148.2438, -24.5) radius 0.5
  circle A1384 centre (-150.7837, -24.5) radius 0.5
  circle A1385 centre (-153.3237, -24.5) radius 0.5
  circle A1386 centre (-155.8638, -24.5) radius 0.5
  circle A1387 centre (-158.4038, -24.5) radius 0.5
  circle A1388 centre (-160.9437, -24.5) radius 0.5
  circle A1389 centre (-163.4838, -24.5) radius 0.5
  circle A1390 centre (-166.0238, -24.5) radius 0.5
  arc A1391 (-175.5625, -20.6375) -> (-175.5625, -19.1375) centre (-175.5625, -19.8875) ccw
  line L728 (-175.5625, -20.6375) -> (-176.8625, -20.6375)
  arc A1392 (-176.8625, -19.1375) -> (-176.8625, -20.6375) centre (-176.8625, -19.8875) ccw
  line L729 (-176.8625, -19.1375) -> (-175.5625, -19.1375)
  circle A1393 centre (-168.5637, -24.5) radius 0.5
  circle A1394 centre (-171.1038, -24.5) radius 0.5
  circle A1395 centre (-173.6438, -24.5) radius 0.5
  circle A1396 centre (-176.1838, -24.5) radius 0.5
  circle A1397 centre (-178.7238, -24.5) radius 0.5
  circle A1398 centre (-181.2637, -24.5) radius 0.5
  circle A1399 centre (-183.8038, -24.5) radius 0.5
  circle A1400 centre (-186.3438, -24.5) radius 0.5
  circle A1401 centre (-186.1138, -30.84) radius 0.5
  circle A1402 centre (-186.1138, -33.38) radius 0.5
  circle A1403 centre (-109.855, -38.1) radius 0.875
  circle A1404 centre (-118.745, -38.1) radius 0.875
  circle A1405 centre (-123.825, -38.1) radius 1.9939
  circle A1406 centre (-120.015, -40.64) radius 1.5
  circle A1407 centre (-128.905, -38.1) radius 0.875
  circle A1408 centre (-126.365, -43.18) radius 1.5
  circle A1409 centre (-138.0838, -42.27) radius 0.5
  circle A1410 centre (-140.6238, -42.28) radius 0.5
  circle A1411 centre (-143.1637, -42.28) radius 0.5
  circle A1412 centre (-145.7038, -42.28) radius 0.5
  circle A1413 centre (-133.35, -47.625) radius 1.1
  circle A1414 centre (-186.1138, -35.92) radius 0.5
  circle A1415 centre (-148.2438, -42.28) radius 0.5
  circle A1416 centre (-150.7837, -42.28) radius 0.5
  circle A1417 centre (-153.3237, -42.28) radius 0.5
  circle A1418 centre (-155.8638, -42.28) radius 0.5
  circle A1419 centre (-158.4038, -42.28) radius 0.5
  circle A1420 centre (-160.9437, -42.28) radius 0.5
  circle A1421 centre (-163.4838, -42.28) radius 0.5
  circle A1422 centre (-166.0238, -42.28) radius 0.5
  circle A1423 centre (-166.0888, -44.3375) radius 0.2
  circle A1424 centre (-166.9487, -44.3375) radius 0.2
  arc A1425 (-165.0988, -45.4875) -> (-164.3987, -45.4875) centre (-164.7488, -45.4875) ccw
  line L730 (-165.0988, -45.4875) -> (-165.0988, -44.1875)
  arc A1426 (-164.3987, -44.1875) -> (-165.0988, -44.1875) centre (-164.7488, -44.1875) ccw
  line L731 (-164.3987, -44.1875) -> (-164.3987, -45.4875)
  circle A1427 centre (-166.0888, -45.6875) radius 0.2
  circle A1428 centre (-166.9487, -45.6875) radius 0.2
  arc A1429 (-165.0988, -49.4275) -> (-164.3987, -49.4275) centre (-164.7488, -49.4275) ccw
  line L732 (-165.0988, -49.4275) -> (-165.0988, -48.5275)
  arc A1430 (-164.3987, -48.5275) -> (-165.0988, -48.5275) centre (-164.7488, -48.5275) ccw
  line L733 (-164.3987, -48.5275) -> (-164.3987, -49.4275)
  circle A1431 centre (-168.5637, -42.28) radius 0.5
  circle A1432 centre (-171.1038, -42.28) radius 0.5
  circle A1433 centre (-173.6438, -42.28) radius 0.5
  circle A1434 centre (-176.1838, -42.28) radius 0.5
  circle A1435 centre (-167.7887, -44.3375) radius 0.2
  circle A1436 centre (-168.6488, -44.3375) radius 0.2
  circle A1437 centre (-169.4888, -44.3375) radius 0.2
  circle A1438 centre (-170.3487, -44.3375) radius 0.2
  circle A1439 centre (-171.1887, -44.3375) radius 0.2
  circle A1440 centre (-167.7887, -45.6875) radius 0.2
  circle A1441 centre (-168.6488, -45.6875) radius 0.2
  circle A1442 centre (-169.4888, -45.6875) radius 0.2
  circle A1443 centre (-170.3487, -45.6875) radius 0.2
  circle A1444 centre (-171.1887, -45.6875) radius 0.2
  circle A1445 centre (-172.0488, -44.3375) radius 0.2
  arc A1446 (-173.7388, -45.4875) -> (-173.0387, -45.4875) centre (-173.3887, -45.4875) ccw
  line L734 (-173.7388, -45.4875) -> (-173.7388, -44.1875)
  arc A1447 (-173.0387, -44.1875) -> (-173.7388, -44.1875) centre (-173.3887, -44.1875) ccw
  line L735 (-173.0387, -44.1875) -> (-173.0387, -45.4875)
  circle A1448 centre (-172.0488, -45.6875) radius 0.2
  circle A1449 centre (-178.7238, -42.28) radius 0.5
  circle A1450 centre (-181.2637, -42.28) radius 0.5
  circle A1451 centre (-183.8038, -42.28) radius 0.5
  circle A1452 centre (-186.3438, -42.28) radius 0.5
  arc A1453 (-173.7388, -49.4275) -> (-173.0387, -49.4275) centre (-173.3887, -49.4275) ccw
  line L736 (-173.7388, -49.4275) -> (-173.7388, -48.5275)
  arc A1454 (-173.0387, -48.5275) -> (-173.7388, -48.5275) centre (-173.3887, -48.5275) ccw
  line L737 (-173.0387, -48.5275) -> (-173.0387, -49.4275)
  circle A1455 centre (-177.3238, -47.625) radius 0.45
  circle A1456 centre (-179.8638, -47.625) radius 0.45
  circle A1457 centre (-185.7375, -47.625) radius 1.1
  circle A1458 centre (128.5875, -47.625) radius 1.1
  circle A1459 centre (107.1563, -47.625) radius 1.1
  circle A1460 centre (26.1938, -47.625) radius 1.1
  circle A1461 centre (-54.7687, -47.625) radius 1.1
  circle A1462 centre (-133.35, -47.625) radius 1.1
  circle A1463 centre (-185.7375, -47.625) radius 1.1
  circle A1464 centre (-161.925, -4.7625) radius 1.1
  circle A1465 centre (-185.7375, 14.2875) radius 1.1
  circle A1466 centre (-161.925, 33.3375) radius 1.1
  circle A1467 centre (-185.7375, 76.2) radius 1.1